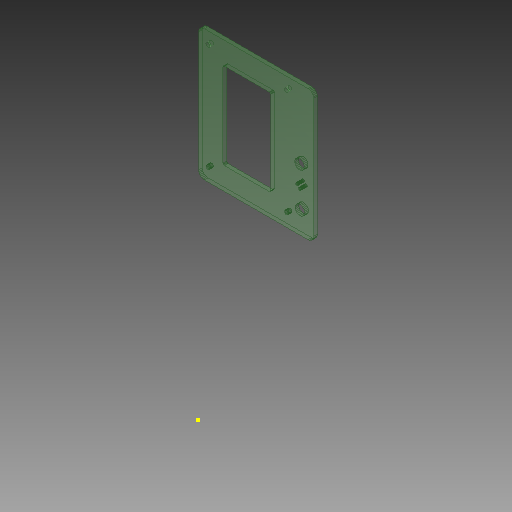
# Autodesk Inventor part: LCD-Front
Saved by Autodesk Inventor 2018 (Build 220112000, 112)
## iProperties
Created: 2016-07-27
Part Number: LCD-Front
Material: Polycarbonate, Green
Document SubType Name: Modeling
Designer: User
Density: 1.2 g/cm^3
Appearance: Polycarbonate - Clear(2)
Mass: 26.5489 g
Surface Area: 169.536 cm^2
Volume: 22.1241 cm^3
Author: User
Autodesk Inventor part; units mm, degrees
ref_plane "YZ Plane" through (0, 0, 0) normal (1, 0, 0) x (0, 1, 0)
ref_plane "XZ Plane" through (0, 0, 0) normal (0, 1, 0) x (-1, 0, 0)
ref_plane "XY Plane" through (0, 0, 0) normal (0, 0, 1) x (1, 0, 0)
sketch "Sketch1" plane through (0, 0, 0) normal (0, 0, 1) x (1, 0, 0)
  line L0 (98.5065, 283.0838) -> (98.1588, 284.0768)
  line L1 (98.1588, 284.0768) -> (97.5989, 284.9679)
  line L2 (97.5989, 284.9679) -> (96.8547, 285.7129)
  line L3 (96.8547, 285.7129) -> (95.9636, 286.273)
  line L4 (95.9636, 286.273) -> (94.9702, 286.62)
  line L5 (94.9702, 286.62) -> (93.9244, 286.738)
  line L6 (93.9244, 286.738) -> (7.9244, 286.738)
  line L7 (7.9244, 286.738) -> (6.8785, 286.62)
  line L8 (6.8785, 286.62) -> (5.8851, 286.273)
  line L9 (5.8851, 286.273) -> (4.994, 285.7131)
  line L10 (4.994, 285.7131) -> (4.2498, 284.9681)
  line L11 (4.2498, 284.9681) -> (3.6898, 284.0771)
  line L12 (3.6898, 284.0771) -> (3.3422, 283.0841)
  line L13 (3.3422, 283.0841) -> (3.2244, 282.0381)
  line L14 (3.2244, 282.0381) -> (3.2244, 182.8381)
  line L15 (3.2244, 182.8381) -> (3.3422, 181.7923)
  line L16 (3.3422, 181.7923) -> (3.6898, 180.7989)
  line L17 (3.6898, 180.7989) -> (4.2498, 179.9077)
  line L18 (4.2498, 179.9077) -> (4.994, 179.1635)
  line L19 (4.994, 179.1635) -> (5.885, 178.6035)
  line L20 (5.885, 178.6035) -> (6.8784, 178.2558)
  line L21 (6.8784, 178.2558) -> (7.9243, 178.1381)
  line L22 (7.9243, 178.1381) -> (93.9243, 178.1381)
  line L23 (93.9243, 178.1381) -> (94.9701, 178.2558)
  line L24 (94.9701, 178.2558) -> (95.9635, 178.6034)
  line L25 (95.9635, 178.6034) -> (96.8546, 179.1634)
  line L26 (96.8546, 179.1634) -> (97.5988, 179.9076)
  line L27 (97.5988, 179.9076) -> (98.1589, 180.7987)
  line L28 (98.1589, 180.7987) -> (98.5066, 181.7921)
  line L29 (98.5066, 181.7921) -> (98.6243, 182.8379)
  line L30 (98.6243, 182.8379) -> (98.6243, 282.0379)
  line L31 (98.6243, 282.0379) -> (98.5065, 283.0838)
  line L32 (62.8881, 267.2996) -> (62.681, 267.7195)
  line L33 (62.681, 267.7195) -> (62.329, 268.0283)
  line L34 (62.329, 268.0283) -> (62.1882, 268.0977)
  line L35 (62.1882, 268.0977) -> (61.729, 268.1891)
  line L36 (61.729, 268.1891) -> (24.6289, 268.1891)
  line L37 (24.6289, 268.1891) -> (24.1697, 268.0977)
  line L38 (24.1697, 268.0977) -> (23.7804, 267.8376)
  line L39 (23.7804, 267.8376) -> (23.5203, 267.4483)
  line L40 (23.5203, 267.4483) -> (23.4289, 266.9891)
  line L41 (23.4289, 266.9891) -> (23.4289, 197.8891)
  line L42 (23.4289, 197.8891) -> (23.5532, 197.4497)
  line L43 (23.5532, 197.4497) -> (23.8168, 197.0769)
  line L44 (23.8168, 197.0769) -> (24.1896, 196.8133)
  line L45 (24.1896, 196.8133) -> (24.6289, 196.6891)
  line L46 (24.6289, 196.6891) -> (61.729, 196.6891)
  line L47 (61.729, 196.6891) -> (62.1882, 196.7804)
  line L48 (62.1882, 196.7804) -> (62.3818, 196.9098)
  line L49 (62.3818, 196.9098) -> (62.5775, 197.0405)
  line L50 (62.5775, 197.0405) -> (62.681, 197.1585)
  line L51 (62.681, 197.1585) -> (62.8881, 197.5785)
  line L52 (62.8881, 197.5785) -> (62.929, 197.8891)
  line L53 (62.929, 197.8891) -> (62.929, 266.989)
  line L54 (62.929, 266.989) -> (62.8881, 267.2996)
  line L55 (90.7765, 229.8734) -> (90.3769, 230.8381)
  line L56 (90.3769, 230.8381) -> (89.7411, 231.6665)
  line L57 (89.7411, 231.6665) -> (88.9127, 232.3022)
  line L58 (88.9127, 232.3022) -> (87.948, 232.7019)
  line L59 (87.948, 232.7019) -> (86.9128, 232.8382)
  line L60 (86.9128, 232.8382) -> (85.8775, 232.7019)
  line L61 (85.8775, 232.7019) -> (84.9128, 232.3023)
  line L62 (84.9128, 232.3023) -> (84.0844, 231.6665)
  line L63 (84.0844, 231.6665) -> (83.4487, 230.8382)
  line L64 (83.4487, 230.8382) -> (83.049, 229.8734)
  line L65 (83.049, 229.8734) -> (82.9127, 228.8382)
  line L66 (82.9127, 228.8382) -> (83.049, 227.8029)
  line L67 (83.049, 227.8029) -> (83.4486, 226.8382)
  line L68 (83.4486, 226.8382) -> (84.0844, 226.0098)
  line L69 (84.0844, 226.0098) -> (84.9127, 225.3741)
  line L70 (84.9127, 225.3741) -> (85.8775, 224.9744)
  line L71 (85.8775, 224.9744) -> (86.9127, 224.8381)
  line L72 (86.9127, 224.8381) -> (87.948, 224.9744)
  line L73 (87.948, 224.9744) -> (88.9127, 225.374)
  line L74 (88.9127, 225.374) -> (89.7411, 226.0098)
  line L75 (89.7411, 226.0098) -> (90.3768, 226.8381)
  line L76 (90.3768, 226.8381) -> (90.7765, 227.8029)
  line L77 (90.7765, 227.8029) -> (90.9127, 228.8383)
  line L78 (90.9127, 228.8383) -> (90.7765, 229.8734)
  line L79 (77.4153, 277.0414) -> (77.4153, 277.0413)
  line L80 (77.4153, 277.0413) -> (77.4261, 277.0152)
  line L81 (77.4261, 277.0152) -> (77.4153, 277.0414)
  line L82 (77.4319, 276.9718) -> (77.4153, 277.0413)
  line L83 (77.4153, 277.0413) -> (77.2713, 277.389)
  line L84 (77.2713, 277.389) -> (77.0249, 277.7101)
  line L85 (77.0249, 277.7101) -> (76.7039, 277.9564)
  line L86 (76.7039, 277.9564) -> (76.3301, 278.1113)
  line L87 (76.3301, 278.1113) -> (75.9289, 278.1641)
  line L88 (75.9289, 278.1641) -> (75.5278, 278.1113)
  line L89 (75.5278, 278.1113) -> (75.1539, 277.9564)
  line L90 (75.1539, 277.9564) -> (74.8329, 277.7101)
  line L91 (74.8329, 277.7101) -> (74.5866, 277.3891)
  line L92 (74.5866, 277.3891) -> (74.4317, 277.0152)
  line L93 (74.4317, 277.0152) -> (74.3789, 276.6141)
  line L94 (74.3789, 276.6141) -> (74.4317, 276.2129)
  line L95 (74.4317, 276.2129) -> (74.5866, 275.8391)
  line L96 (74.5866, 275.8391) -> (74.8957, 275.47)
  line L97 (74.8957, 275.47) -> (74.8329, 275.5181)
  line L98 (74.8329, 275.5181) -> (75.1245, 275.2943)
  line L99 (75.1245, 275.2943) -> (75.1539, 275.2718)
  line L100 (75.1539, 275.2718) -> (75.4324, 275.1564)
  line L101 (75.4324, 275.1564) -> (75.5278, 275.1169)
  line L102 (75.5278, 275.1169) -> (75.6583, 275.0997)
  line L103 (75.6583, 275.0997) -> (75.9289, 275.0641)
  line L104 (75.9289, 275.0641) -> (76.3301, 275.1169)
  line L105 (76.3301, 275.1169) -> (76.7039, 275.2718)
  line L106 (76.7039, 275.2718) -> (77.0249, 275.5181)
  line L107 (77.0249, 275.5181) -> (77.2713, 275.8391)
  line L108 (77.2713, 275.8391) -> (77.4261, 276.2129)
  line L109 (77.4261, 276.2129) -> (77.4537, 276.4224)
  line L110 (77.4537, 276.4224) -> (77.4652, 276.719)
  line L111 (77.4652, 276.719) -> (77.4319, 276.9718)
  line L112 (77.4261, 189.0653) -> (77.2712, 189.4391)
  line L113 (77.2712, 189.4391) -> (77.0249, 189.7601)
  line L114 (77.0249, 189.7601) -> (76.7039, 190.0064)
  line L115 (76.7039, 190.0064) -> (76.33, 190.1613)
  line L116 (76.33, 190.1613) -> (75.9289, 190.2141)
  line L117 (75.9289, 190.2141) -> (75.5277, 190.1613)
  line L118 (75.5277, 190.1613) -> (75.0743, 189.9453)
  line L119 (75.0743, 189.9453) -> (74.7753, 189.6851)
  line L120 (74.7753, 189.6851) -> (74.6174, 189.4793)
  line L121 (74.6174, 189.4793) -> (74.4317, 189.0653)
  line L122 (74.4317, 189.0653) -> (74.3789, 188.6641)
  line L123 (74.3789, 188.6641) -> (74.4317, 188.2629)
  line L124 (74.4317, 188.2629) -> (74.5866, 187.8891)
  line L125 (74.5866, 187.8891) -> (74.8329, 187.5681)
  line L126 (74.8329, 187.5681) -> (75.154, 187.3217)
  line L127 (75.154, 187.3217) -> (75.5278, 187.1669)
  line L128 (75.5278, 187.1669) -> (75.9289, 187.1141)
  line L129 (75.9289, 187.1141) -> (76.3301, 187.1669)
  line L130 (76.3301, 187.1669) -> (76.7039, 187.3217)
  line L131 (76.7039, 187.3217) -> (77.025, 187.5681)
  line L132 (77.025, 187.5681) -> (77.2817, 187.9143)
  line L133 (77.2817, 187.9143) -> (77.3677, 188.1219)
  line L134 (77.3677, 188.1219) -> (77.4261, 188.2629)
  line L135 (77.4261, 188.2629) -> (77.4516, 188.4563)
  line L136 (77.4516, 188.4563) -> (77.4789, 188.6641)
  line L137 (77.4789, 188.6641) -> (77.4261, 189.0653)
  line L138 (12.4262, 189.0652) -> (12.2713, 189.439)
  line L139 (12.2713, 189.439) -> (12.1053, 189.6554)
  line L140 (12.1053, 189.6554) -> (12.025, 189.76)
  line L141 (12.025, 189.76) -> (11.704, 190.0063)
  line L142 (11.704, 190.0063) -> (11.3302, 190.1612)
  line L143 (11.3302, 190.1612) -> (10.929, 190.214)
  line L144 (10.929, 190.214) -> (10.5278, 190.1612)
  line L145 (10.5278, 190.1612) -> (10.2066, 190.0064)
  line L146 (10.2066, 190.0064) -> (9.9709, 189.8659)
  line L147 (9.9709, 189.8659) -> (9.833, 189.7601)
  line L148 (9.833, 189.7601) -> (9.5866, 189.4391)
  line L149 (9.5866, 189.4391) -> (9.4318, 189.0652)
  line L150 (9.4318, 189.0652) -> (9.379, 188.6641)
  line L151 (9.379, 188.6641) -> (9.4318, 188.2629)
  line L152 (9.4318, 188.2629) -> (9.5866, 187.8891)
  line L153 (9.5866, 187.8891) -> (9.833, 187.5681)
  line L154 (9.833, 187.5681) -> (10.154, 187.3217)
  line L155 (10.154, 187.3217) -> (10.5278, 187.1669)
  line L156 (10.5278, 187.1669) -> (10.6106, 187.1778)
  line L157 (10.6106, 187.1778) -> (10.929, 187.114)
  line L158 (10.929, 187.114) -> (11.3301, 187.1668)
  line L159 (11.3301, 187.1668) -> (11.7039, 187.3217)
  line L160 (11.7039, 187.3217) -> (12.025, 187.5681)
  line L161 (12.025, 187.5681) -> (12.2713, 187.889)
  line L162 (12.2713, 187.889) -> (12.4261, 188.2629)
  line L163 (12.4261, 188.2629) -> (12.479, 188.6641)
  line L164 (12.479, 188.6641) -> (12.4262, 189.0652)
  line L165 (87.8787, 211.2664) -> (87.7788, 211.5076)
  line L166 (87.7788, 211.5076) -> (87.6198, 211.7146)
  line L167 (87.6198, 211.7146) -> (87.4127, 211.8736)
  line L168 (87.4127, 211.8736) -> (87.1716, 211.9735)
  line L169 (87.1716, 211.9735) -> (86.9127, 212.0075)
  line L170 (86.9127, 212.0075) -> (86.654, 211.9735)
  line L171 (86.654, 211.9735) -> (86.4128, 211.8736)
  line L172 (86.4128, 211.8736) -> (86.2056, 211.7146)
  line L173 (86.2056, 211.7146) -> (86.0467, 211.5076)
  line L174 (86.0467, 211.5076) -> (85.9468, 211.2664)
  line L175 (85.9468, 211.2664) -> (85.9128, 211.0076)
  line L176 (85.9128, 211.0076) -> (85.9468, 210.7488)
  line L177 (85.9468, 210.7488) -> (86.0468, 210.5076)
  line L178 (86.0468, 210.5076) -> (86.2057, 210.3005)
  line L179 (86.2057, 210.3005) -> (86.4127, 210.1416)
  line L180 (86.4127, 210.1416) -> (86.6539, 210.0417)
  line L181 (86.6539, 210.0417) -> (86.9127, 210.0076)
  line L182 (86.9127, 210.0076) -> (87.1716, 210.0417)
  line L183 (87.1716, 210.0417) -> (87.4127, 210.1415)
  line L184 (87.4127, 210.1415) -> (87.6198, 210.3005)
  line L185 (87.6198, 210.3005) -> (87.7787, 210.5075)
  line L186 (87.7787, 210.5075) -> (87.8786, 210.7488)
  line L187 (87.8786, 210.7488) -> (87.9127, 211.0077)
  line L188 (87.9127, 211.0077) -> (87.8787, 211.2664)
  line L189 (85.5381, 213.6068) -> (85.4381, 213.8481)
  line L190 (85.4381, 213.8481) -> (85.2792, 214.0551)
  line L191 (85.2792, 214.0551) -> (85.0722, 214.214)
  line L192 (85.0722, 214.214) -> (84.8309, 214.314)
  line L193 (84.8309, 214.314) -> (84.5722, 214.348)
  line L194 (84.5722, 214.348) -> (84.3133, 214.314)
  line L195 (84.3133, 214.314) -> (84.0722, 214.2141)
  line L196 (84.0722, 214.2141) -> (83.8651, 214.0553)
  line L197 (83.8651, 214.0553) -> (83.7061, 213.8482)
  line L198 (83.7061, 213.8482) -> (83.6063, 213.6069)
  line L199 (83.6063, 213.6069) -> (83.5723, 213.3482)
  line L200 (83.5723, 213.3482) -> (83.6062, 213.0894)
  line L201 (83.6062, 213.0894) -> (83.7062, 212.8482)
  line L202 (83.7062, 212.8482) -> (83.8651, 212.6411)
  line L203 (83.8651, 212.6411) -> (84.0722, 212.4821)
  line L204 (84.0722, 212.4821) -> (84.3133, 212.3822)
  line L205 (84.3133, 212.3822) -> (84.5722, 212.3482)
  line L206 (84.5722, 212.3482) -> (84.831, 212.3822)
  line L207 (84.831, 212.3822) -> (85.0722, 212.4821)
  line L208 (85.0722, 212.4821) -> (85.2793, 212.641)
  line L209 (85.2793, 212.641) -> (85.4382, 212.8481)
  line L210 (85.4382, 212.8481) -> (85.5381, 213.0893)
  line L211 (85.5381, 213.0893) -> (85.5721, 213.3479)
  line L212 (85.5721, 213.3479) -> (85.5381, 213.6068)
  line L213 (87.8787, 215.9474) -> (87.7788, 216.1887)
  line L214 (87.7788, 216.1887) -> (87.6199, 216.3957)
  line L215 (87.6199, 216.3957) -> (87.4128, 216.5547)
  line L216 (87.4128, 216.5547) -> (87.1716, 216.6546)
  line L217 (87.1716, 216.6546) -> (86.9128, 216.6886)
  line L218 (86.9128, 216.6886) -> (86.654, 216.6546)
  line L219 (86.654, 216.6546) -> (86.4128, 216.5547)
  line L220 (86.4128, 216.5547) -> (86.2057, 216.3957)
  line L221 (86.2057, 216.3957) -> (86.0468, 216.1887)
  line L222 (86.0468, 216.1887) -> (85.9468, 215.9475)
  line L223 (85.9468, 215.9475) -> (85.9128, 215.6887)
  line L224 (85.9128, 215.6887) -> (85.9468, 215.4299)
  line L225 (85.9468, 215.4299) -> (86.0467, 215.1887)
  line L226 (86.0467, 215.1887) -> (86.2056, 214.9816)
  line L227 (86.2056, 214.9816) -> (86.4128, 214.8227)
  line L228 (86.4128, 214.8227) -> (86.6539, 214.7227)
  line L229 (86.6539, 214.7227) -> (86.9127, 214.6887)
  line L230 (86.9127, 214.6887) -> (87.1716, 214.7227)
  line L231 (87.1716, 214.7227) -> (87.4127, 214.8227)
  line L232 (87.4127, 214.8227) -> (87.6198, 214.9816)
  line L233 (87.6198, 214.9816) -> (87.7788, 215.1887)
  line L234 (87.7788, 215.1887) -> (87.8787, 215.4299)
  line L235 (87.8787, 215.4299) -> (87.9128, 215.6889)
  line L236 (87.9128, 215.6889) -> (87.8787, 215.9474)
  line L237 (91.1427, 197.1234) -> (90.7431, 198.0881)
  line L238 (90.7431, 198.0881) -> (90.1074, 198.9165)
  line L239 (90.1074, 198.9165) -> (89.279, 199.5522)
  line L240 (89.279, 199.5522) -> (88.3143, 199.9519)
  line L241 (88.3143, 199.9519) -> (87.279, 200.0882)
  line L242 (87.279, 200.0882) -> (86.2437, 199.9519)
  line L243 (86.2437, 199.9519) -> (85.279, 199.5523)
  line L244 (85.279, 199.5523) -> (84.4506, 198.9165)
  line L245 (84.4506, 198.9165) -> (83.8149, 198.0881)
  line L246 (83.8149, 198.0881) -> (83.4152, 197.1234)
  line L247 (83.4152, 197.1234) -> (83.2789, 196.0882)
  line L248 (83.2789, 196.0882) -> (83.4152, 195.0528)
  line L249 (83.4152, 195.0528) -> (83.8148, 194.0882)
  line L250 (83.8148, 194.0882) -> (84.4506, 193.2598)
  line L251 (84.4506, 193.2598) -> (85.279, 192.624)
  line L252 (85.279, 192.624) -> (86.2437, 192.2244)
  line L253 (86.2437, 192.2244) -> (87.2789, 192.0881)
  line L254 (87.2789, 192.0881) -> (88.3139, 192.2244)
  line L255 (88.3139, 192.2244) -> (89.2786, 192.624)
  line L256 (89.2786, 192.624) -> (90.1069, 193.2597)
  line L257 (90.1069, 193.2597) -> (90.7427, 194.0881)
  line L258 (90.7427, 194.0881) -> (91.1423, 195.0528)
  line L259 (91.1423, 195.0528) -> (91.2788, 196.0896)
  line L260 (91.2788, 196.0896) -> (91.1427, 197.1234)
  line L261 (90.2238, 213.6073) -> (90.1238, 213.8486)
  line L262 (90.1238, 213.8486) -> (89.9649, 214.0557)
  line L263 (89.9649, 214.0557) -> (89.7578, 214.2146)
  line L264 (89.7578, 214.2146) -> (89.5167, 214.3145)
  line L265 (89.5167, 214.3145) -> (89.2579, 214.3486)
  line L266 (89.2579, 214.3486) -> (88.999, 214.3145)
  line L267 (88.999, 214.3145) -> (88.7579, 214.2147)
  line L268 (88.7579, 214.2147) -> (88.5509, 214.0557)
  line L269 (88.5509, 214.0557) -> (88.3918, 213.8488)
  line L270 (88.3918, 213.8488) -> (88.2919, 213.6075)
  line L271 (88.2919, 213.6075) -> (88.2579, 213.3487)
  line L272 (88.2579, 213.3487) -> (88.2918, 213.09)
  line L273 (88.2918, 213.09) -> (88.3918, 212.8488)
  line L274 (88.3918, 212.8488) -> (88.5508, 212.6417)
  line L275 (88.5508, 212.6417) -> (88.7579, 212.4827)
  line L276 (88.7579, 212.4827) -> (88.999, 212.3829)
  line L277 (88.999, 212.3829) -> (89.2579, 212.3488)
  line L278 (89.2579, 212.3488) -> (89.5167, 212.3828)
  line L279 (89.5167, 212.3828) -> (89.7578, 212.4827)
  line L280 (89.7578, 212.4827) -> (89.9649, 212.6417)
  line L281 (89.9649, 212.6417) -> (90.1238, 212.8488)
  line L282 (90.1238, 212.8488) -> (90.2238, 213.09)
  line L283 (90.2238, 213.09) -> (90.2578, 213.3487)
  line L284 (90.2578, 213.3487) -> (90.2238, 213.6073)
  line L285 (12.4262, 277.0152) -> (12.2713, 277.389)
  line L286 (12.2713, 277.389) -> (12.025, 277.71)
  line L287 (12.025, 277.71) -> (11.704, 277.9564)
  line L288 (11.704, 277.9564) -> (11.3301, 278.1113)
  line L289 (11.3301, 278.1113) -> (10.929, 278.1641)
  line L290 (10.929, 278.1641) -> (10.5278, 278.1112)
  line L291 (10.5278, 278.1112) -> (10.154, 277.9564)
  line L292 (10.154, 277.9564) -> (9.833, 277.7101)
  line L293 (9.833, 277.7101) -> (9.5866, 277.389)
  line L294 (9.5866, 277.389) -> (9.4318, 277.0152)
  line L295 (9.4318, 277.0152) -> (9.379, 276.6141)
  line L296 (9.379, 276.6141) -> (9.4318, 276.2129)
  line L297 (9.4318, 276.2129) -> (9.5866, 275.8391)
  line L298 (9.5866, 275.8391) -> (9.833, 275.5181)
  line L299 (9.833, 275.5181) -> (10.154, 275.2717)
  line L300 (10.154, 275.2717) -> (10.5278, 275.1169)
  line L301 (10.5278, 275.1169) -> (10.929, 275.0641)
  line L302 (10.929, 275.0641) -> (11.3301, 275.1169)
  line L303 (11.3301, 275.1169) -> (11.704, 275.2717)
  line L304 (11.704, 275.2717) -> (12.025, 275.5181)
  line L305 (12.025, 275.5181) -> (12.2713, 275.8391)
  line L306 (12.2713, 275.8391) -> (12.4262, 276.2129)
  line L307 (12.4262, 276.2129) -> (12.479, 276.6141)
  line L308 (12.479, 276.6141) -> (12.4262, 277.0152)
  point P0 (0, 0)
  constraints: 618 end point, 17 parallel, 17 perpendicular, 1 collinear
extrude "Extrusion1" add sketch "Sketch1" along normal blind 3 contours L31 L30 L29 L28 L27 L26 L25 L24 L23 L22 L21 L20 L19 L18 L17 L16 L15 L14 L13 L12 L11 L10 L9 L8 L7 L6 L5 L4 L3 L2 L1 L0 | L111 L110 L109 L108 L107 L106 L105 L104 L103 L102 L101 L100 L99 L98 L96 L95 L94 L93 L92 L91 L90 L89 L88 L87 L86 L85 L84 L83 L82
sketch "Sketch2" plane through (0, 0, 0) normal (0, 0, -1) x (-1, 0, 0)
  line L0 (-9.4318, 276.2129) -> (-9.379, 276.6141) projected
  line L1 (-9.379, 276.6141) -> (-12.4794, 276.6141)
  circle A0 centre (-10.9292, 276.6141) radius 1.7
  point P0 (0, 0)
  dimension "d2" = 3.4
  constraints: 2 end point, 1 centre point, 1 horizontal, 1 midpoint
  measures "d2" diameter of A0
extrude "Extrusion2" cut sketch "Sketch2" against normal blind 3
sketch "Sketch3" plane through (0, 0, 0) normal (0, 0, -1) x (-1, 0, 0)
  circle A0 centre (-75.9292, 276.6141) radius 1.55 projected
  point P0 (0, 0)
extrude "Extrusion3" cut sketch "Sketch3" against normal blind 10
sketch "Sketch4" plane through (0, 0, 0) normal (0, 0, -1) x (-1, 0, 0)
  point P0 (0, 0)
body "Solid1"
